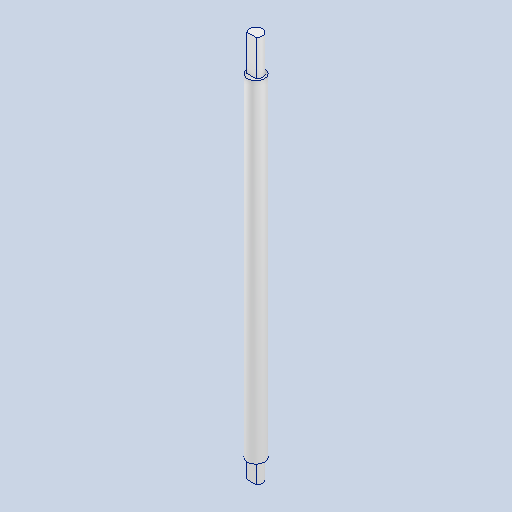
# Autodesk Inventor part: screw_screw
Saved by Autodesk Inventor 2024.1 (Build 281209000, 209)
## iProperties
Created: 2025-01-17
Part Number: screw_screw
Material: アルミニウム 6061
Document SubType Name: Modeling
Designer: hibik
Density: 2.7 g/cm^3
Appearance: アルミニウム - フラット
Author: hibik
Autodesk Inventor part; units mm, degrees
ref_plane "YZ Plane" through (0, 0, 0) normal (1, 0, 0) x (0, 1, 0)
ref_plane "XZ Plane" through (0, 0, 0) normal (0, 1, 0) x (-1, 0, 0)
ref_plane "XY Plane" through (0, 0, 0) normal (0, 0, 1) x (1, 0, 0)
sketch "スケッチ1" plane through (0, 0, 0) normal (0, 1, 0) x (-1, 0, 0)
  circle A0 centre (0, 0) radius 2
  dimension "d0" = 4
  constraints: 1 centre point, 1 coincident
  measures "d0" diameter of A0
extrude "押し出し1" add sketch "スケッチ1" along normal blind 97
sketch "スケッチ2" plane through (0, 0, 0) normal (0, -1, 0) x (1, 0, 0)
  circle A0 centre (0, 0) radius 1.5
  line L0 (-1.118, 1) -> (1.118, 1)
  circle A1 centre (0, 0) radius 2 projected
  circle A2 centre (0, 0) radius 2 projected
  dimension "d3" = 3
  dimension "d4" = 1
  constraints: 2 end point, 2 point on circle, 1 centre point, 1 coincident, 1 horizontal
  measures "d3" diameter of A0
  measures "d4" distance from line of point (0, 0) L0
extrude "押し出し2" cut sketch "スケッチ2" against normal blind 8 contours L0 A0 | A1 picked at (-0.0599, 1.1631)
sketch "スケッチ3" plane through (0, 97, 0) normal (0, 1, 0) x (1, 0, 0)
  arc A0 (1.118, -1) -> (-1.118, -1) centre (0, 0) ccw projected
  line L0 (1.118, -1) -> (-1.118, -1) projected
  circle A1 centre (0, 0) radius 2 projected
extrude "押し出し3" cut sketch "スケッチ3" against normal blind 12
sketch "スケッチ4" plane through (0, 97, 0) normal (0, 1, 0) x (1, 0, 0)
  arc A0 (1.118, -1) -> (-1.118, -1) centre (0, 0) ccw projected
  line L0 (-1.118, -1) -> (1.118, -1) projected
extrude "押し出し4" cut sketch "スケッチ4" against normal blind 3.7
sketch "スケッチ5" plane through (0, 0, 0) normal (0, -1, 0) x (1, 0, 0)
  line L0 (1.118, 1) -> (-1.118, 1) projected
  arc A0 (-1.118, 1) -> (1.118, 1) centre (0, 0) ccw projected
extrude "押し出し5" cut sketch "スケッチ5" against normal blind 3.5
